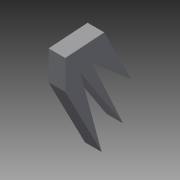
# Autodesk Inventor part: ring1_rollerFace_JacobMorgan_030515_pd3
Saved by Autodesk Inventor 2015 (Build 190159000, 159)
## iProperties
Created: 2015-03-05
Part Number: ring1_rollerFace_JacobMorgan_030515_pd3
Material: Generic
Document SubType Name: Modeling
Designer: WASHHSST
Density: 1 g/cm^3
Appearance: Default
Author: WASHHSST
Autodesk Inventor part; units mm, degrees
ref_plane "YZ Plane" through (0, 0, 0) normal (1, 0, 0) x (0, 1, 0)
ref_plane "XZ Plane" through (0, 0, 0) normal (0, 1, 0) x (-1, 0, 0)
ref_plane "XY Plane" through (0, 0, 0) normal (0, 0, 1) x (1, 0, 0)
sketch "Sketch1" plane through (0, 0, 0) normal (1, 0, 0) x (0, 1, 0)
  line L0 (2.0163, 3.3983) -> (6.5021, 3.3983)
  line L1 (6.5021, 3.3983) -> (6.9099, -2.5374)
  line L2 (6.9099, -2.5374) -> (-1.3367, -6.6607)
  line L3 (-1.3367, -6.6607) -> (3.8287, -0.6343)
  line L4 (3.8287, -0.6343) -> (-6.5021, -5.392)
  line L5 (-6.5021, -5.392) -> (3.4663, 1.1328)
  line L6 (3.4663, 1.1328) -> (-8.6374, -2.1296)
  line L7 (-8.6374, -2.1296) -> (2.0163, 3.3983)
  point P0 (0, 0)
  constraints: 16 end point, 1 horizontal
extrude "Extrusion2" add sketch "Sketch1" along normal blind 2.54
body "Solid2"
